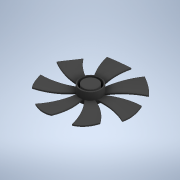
# Autodesk Inventor part: Pc Fan 120 mm - fan
Saved by Autodesk Inventor 2020 (Build 240168000, 168)
## iProperties
Created: 2021-05-19
Part Number: Pc Fan 120 mm - fan
Material: Generic
Document SubType Name: Modeling
Designer: 6128059
Density: 1 g/cm^3
Appearance: Default
Author: 6128059
Autodesk Inventor part; units mm, degrees
ref_plane "XY Plane" through (0, 0, 0) normal (0, 0, 1) x (1, 0, 0)
sketch "Sketch1" plane through (0, 0, 0) normal (0, 1, 0) x (-1, 0, 0)
  circle A0 centre (0, 0) radius 12.5
  circle A1 centre (0, 0) radius 55
  dimension "d0" = 25
  dimension "d1" = 110
  constraints: 2 centre point, 2 coincident
  measures "d0" diameter of A0
  measures "d1" diameter of A1
extrude "Extrusion1" add sketch "Sketch1" along normal blind 20
sketch "Sketch2" plane through (0, 20, 0) normal (0, 1, 0) x (1, 0, 0)
  circle A0 centre (0, 0) radius 55 projected
  circle A1 centre (0, 0) radius 12.5 projected
  arc A2 (52.915, 15) -> (11.4564, 5) centre (49.046, -59.9001) ccw
  arc A3 (53.6749, -12) -> (11.4564, -5) centre (20.8077, -79.4147) ccw
  dimension "d4" = 5
  dimension "d5" = 5
  dimension "d6" = 75
  dimension "d7" = 75
  dimension "d8" = 15
  dimension "d9" = 12
  constraints: 8 point on circle, 2 centre point
  measures "d4" vertical distance of A0.centre A1.end
  measures "d5" vertical distance of A1.start A0.centre
  measures "d6" radius of A3
  measures "d7" radius of A2
  measures "d8" vertical distance of A0.centre A0.start
  measures "d9" vertical distance of A0.centre A0.end
extrude "Extrusion2" cut sketch "Sketch2" against normal blind 20 contours A2 A1 A3 A0 picked at (18.2843, 22.7058)
ref_plane "Work Plane1" through (55, 0, 0) normal (1, 0, 0) x (0, 1, 0)
sketch "Sketch3" plane through (55, 0, 0) normal (1, 0, 0) x (0, 1, 0)
  line L0 (0, -15) -> (20, -15) projected
  line L1 (20, 12) -> (20, -15) projected
  line L2 (20, 12) -> (0, 12) projected
  line L3 (0, 12) -> (0, -15) projected
  line L4 (20, 12) -> (0, 12) projected
  arc A0 (10, 12) -> (13.5, -15) centre (84.8923, 7.9814) ccw
  line L5 (0, -15) -> (20, -15) projected
  arc A1 (8.5, 12) -> (12, -15) centre (83.3923, 7.9814) ccw
  point P0 (0, 0)
  point P1 (12, -15)
  point P2 (10, 12)
  dimension "d13" = 75
  dimension "d14" = 1.5
  dimension "d15" = 1.5
  dimension "d16" = 2
  constraints: 4 point on circle, 3 point on line, 2 centre point, 1 equal radius, 1 midpoint
  measures "d13" radius of A1
  measures "d14" distance of A0.start A1.start
  measures "d15" distance of A1.end A0.end
  measures "d16" horizontal distance of A0.start A1.end
sketch3d "3D Sketch2"
  arc A0 (53.6749, 20, 12) -> (11.4564, 20, 5) centre (20.8077, 20, 79.4147) ccw
sweep "Sweep1" cut profiles "Sketch3" path "3D Sketch2" keep common part contours A1 L2 A0 L0
pattern_circular "Circular Pattern1" count 7 over 360 about axis through (0, -10, 0) along (0, 1, 0)
ref_plane "Work Plane2" through (0, 5, 0) normal (0, 1, 0) x (-1, 0, 0)
sketch "Sketch4" plane through (0, 5, 0) normal (0, 1, 0) x (-1, 0, 0)
  circle A0 centre (0, 0) radius 14
  point P0 (2.0672, 13.8465)
  point P1 (10.0402, 9.7568)
  dimension "d25" = 28
  constraints: 1 centre point, 1 coincident, 1 other
  measures "d25" diameter of A0
extrude "Extrusion3" add sketch "Sketch4" along normal blind 15
sketch "Sketch5" plane through (0, 20, 0) normal (0, 1, 0) x (1, 0, 0)
  circle A0 centre (0, 0) radius 12.5
  dimension "d26" = 25
  constraints: 1 centre point, 1 coincident
  measures "d26" diameter of A0
extrude "Extrusion4" cut sketch "Sketch5" against normal blind 12
sketch "Sketch6" plane through (0, 8, 0) normal (0, 1, 0) x (1, 0, 0)
  circle A0 centre (0, 0) radius 10
  dimension "d29" = 20
  constraints: 1 centre point, 1 coincident
  measures "d29" diameter of A0
extrude "Extrusion5" add sketch "Sketch6" along normal blind 12
sketch "Sketch7" plane through (0, 5, 0) normal (0, -1, 0) x (1, 0, 0)
  line L0 (-10, -18) -> (-10, 18) construction
  line L1 (-10, 18) -> (10, 18) construction
  line L2 (10, 18) -> (10, -18) construction
  line L3 (10, -18) -> (-10, -18) construction
  line L4 (-8.3031, 0.4567) -> (-7.4264, 1.7434)
  line L5 (-7.4264, 1.7434) -> (-6.8352, 2.528)
  arc A0 (-4.8118, 4.6535) -> (-6.8352, 2.528) centre (3.3814, -5.1717) ccw
  arc A1 (-3.1565, 5.6276) -> (-4.8118, 4.6535) centre (-1.0264, 0.1141) ccw
  arc A2 (-1.2858, 5.6808) -> (-3.1565, 5.6276) centre (-2.1459, 3.0117) ccw
  arc A3 (-1.2858, 5.6808) -> (-1.7353, 5.5258) centre (-1.0185, 4.1769) ccw
  arc A4 (-1.7353, 5.5258) -> (-2.7655, 4.6462) centre (-0.2675, 2.7636) ccw
  line L6 (-2.7655, 4.6462) -> (-3.2359, 4.022)
  arc A5 (-3.2359, 4.022) -> (-3.4458, 3.6894) centre (-1.3384, 2.592) ccw
  line L7 (-3.4458, 3.6894) -> (-3.8181, 2.9744)
  line L8 (-3.8181, 2.9744) -> (-4.1655, 2.1067)
  arc A6 (-4.1655, 2.1067) -> (-4.9023, 2.07) centre (-4.4435, 0.2769) ccw
  arc A7 (-4.9023, 2.07) -> (-5.9084, 1.7079) centre (-3.5044, -3.3934) ccw
  arc A8 (-5.9084, 1.7079) -> (-8.3031, 0.4567) centre (3.3917, -19.0085) ccw
  line L9 (-5.8142, -2.8999) -> (-4.1655, -0.5885)
  arc A9 (-3.6087, -0.3916) -> (-4.1655, -0.5885) centre (-3.2244, -2.364) ccw
  line L10 (-3.6087, -0.3916) -> (-1.6961, -0.0191)
  line L11 (-1.6961, -0.0191) -> (-2.7283, -2.0606)
  arc A10 (-2.7283, -2.0606) -> (-3.9473, -2.1696) centre (-2.955, -6.3971) ccw
  arc A11 (-3.9473, -2.1696) -> (-5.0366, -2.5317) centre (-1.2206, -12.1916) ccw
  arc A12 (-5.0366, -2.5317) -> (-5.8142, -2.8999) centre (-2.6419, -8.5937) ccw
  line L12 (-3.722, -6.6222) -> (-2.506, -4.3734)
  arc A13 (-0.4573, -3.7848) -> (-2.506, -4.3734) centre (2.5217, -18.0142) ccw
  line L13 (-0.4573, -3.7848) -> (-1.2689, -5.39)
  arc A14 (-1.2689, -5.39) -> (-2.3841, -5.7728) centre (-0.3459, -9.8948) ccw
  arc A15 (-2.3841, -5.7728) -> (-3.722, -6.6222) centre (0.9225, -12.4598) ccw
  line L14 (0.8426, -3.3597) -> (-1.2206, -7.0503)
  arc A16 (1.0045, -6.3391) -> (-1.2206, -7.0503) centre (2.6736, -15.3978) ccw
  arc A17 (7.9001, -8.3008) -> (1.0045, -6.3391) centre (2.4695, -14.2898) ccw
  line L15 (7.9001, -8.3008) -> (6.5614, -4.7114)
  arc A18 (4.6829, 2.7002) -> (6.5614, -4.7114) centre (39.567, 7.5979) ccw
  arc A19 (4.6265, 5.3315) -> (4.6829, 2.7002) centre (15.7497, 4.2539) ccw
  arc A20 (4.9549, 6.5803) -> (4.6265, 5.3315) centre (8.645, 4.9422) ccw
  arc A21 (5.8182, 7.4988) -> (4.9549, 6.5803) centre (6.699, 5.8061) ccw
  arc A22 (5.8182, 7.4988) -> (3.9321, 8.2911) centre (3.2793, 4.096) ccw
  arc A23 (3.9321, 8.2911) -> (2.5001, 8.1608) centre (3.421, 5.9743) ccw
  arc A24 (2.5001, 8.1608) -> (1.7356, 7.7143) centre (3.8256, 5.0138) ccw
  line L16 (-5.3722, -0.3769) -> (-3.5044, 2.07)
  line L17 (-3.5044, 2.07) -> (-1.378, 4.6029)
  line L18 (-1.378, 4.6029) -> (-0.35, 5.7629)
  arc A25 (1.7356, 7.7143) -> (-0.35, 5.7629) centre (11.0968, -4.3814) ccw
  arc A26 (-3.8943, 0.4313) -> (-5.3722, -0.3769) centre (5.3947, -18.3109) ccw
  arc A27 (-1.5445, 1.229) -> (-3.8943, 0.4313) centre (-0.4186, -5.9474) ccw
  arc A28 (0.7074, 1.229) -> (-1.5445, 1.229) centre (-0.4186, -5.9474) ccw
  arc A29 (4.5034, -0.1136) -> (0.7074, 1.229) centre (-1.1856, -10.1607) ccw
  arc A30 (4.5034, -0.1136) -> (-0.3792, 0.3979) centre (0.6046, -13.7718) ccw
  line L19 (-0.3792, 0.3979) -> (-2.8956, -3.7347)
  arc A31 (5.2344, -3.6297) -> (-2.8956, -3.7347) centre (1.2719, -11.623) ccw
  arc A32 (5.2344, -3.6297) -> (0.8426, -3.3597) centre (1.9323, -21.4832) ccw
  point P0 (0, 0)
  point P1 (0, 18)
  point P2 (-10, 0)
  dimension "d36" = 20
  constraints: 66 point on circle, 33 centre point, 32 end point, 19 tangent, 2 midpoint, 1 horizontal alignment, 1 vertical, 1 vertical alignment, 51 other
  measures "d36" distance of L0.end L1.end
extrude "Extrusion6" cut sketch "Sketch7" against normal blind 0.5
body "Solid1"
